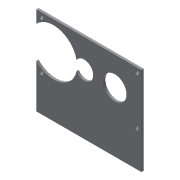
# Autodesk Inventor part: attatching plate for toughbox
Saved by Autodesk Inventor 2015 (Build 190159000, 159)
## iProperties
Created: 2015-02-15
Part Number: attatching plate for toughbox
Material: Generic
Document SubType Name: Sheet Metal
Designer: Noah
Density: 1 g/cm^3
Sheet Metal Rule: Default
Appearance: Default
Author: Noah
Autodesk Inventor part; units mm, degrees
ref_plane "YZ Plane" through (0, 0, 0) normal (1, 0, 0) x (0, 1, 0)
ref_plane "XZ Plane" through (0, 0, 0) normal (0, 1, 0) x (-1, 0, 0)
ref_plane "XY Plane" through (0, 0, 0) normal (0, 0, 1) x (1, 0, 0)
sketch "Sketch1" plane through (0, 0, 0) normal (0, 0, 1) x (1, 0, 0)
  line L0 (0, 0) -> (139.7, 0)
  line L1 (139.7, 0) -> (139.7, 117.475)
  line L2 (139.7, 117.475) -> (0, 117.475)
  line L3 (0, 117.475) -> (0, 0)
  dimension "d0" = 139.7
  dimension "d1" = 117.475
  measures "d0" distance of L2.end L1.end
  measures "d1" distance of L0.end L1.end
extrude "Plate3" add sketch "Sketch1" along normal blind 3.048
sketch "Sketch4" plane through (0, 0, 0) normal (0, 0, -1) x (-1, 0, 0)
  circle A0 centre (-22.86, 79.375) radius 31.242
  circle A1 centre (-6.35, 111.125) radius 2.5527
  circle A2 centre (-6.35, 47.625) radius 2.5527
  circle A3 centre (-133.35, 111.125) radius 2.5527
  circle A4 centre (-133.35, 47.625) radius 2.5527
  arc A5 (-136.4869, 13.4874) -> (-136.4869, 27.7876) centre (-136.4869, 20.6375) ccw
  line L0 (-150.7617, 27.7876) -> (-136.4869, 27.7876)
  line L1 (-136.4869, 13.4874) -> (-150.7617, 13.4874)
  arc A6 (-99.9617, 27.7876) -> (-99.9617, 13.4874) centre (-99.9617, 20.6375) ccw
  line L2 (-99.9617, 27.7876) -> (-85.6869, 27.7876)
  line L3 (-85.6869, 13.4874) -> (-99.9617, 13.4874)
  arc A7 (-85.6869, 13.4874) -> (-85.6869, 27.7876) centre (-85.6869, 20.6375) ccw
  arc A8 (-49.1617, 27.7876) -> (-49.1617, 13.4874) centre (-49.1617, 20.6375) ccw
  line L4 (-49.1617, 27.7876) -> (-34.8869, 27.7876)
  arc A9 (-34.8869, 13.4874) -> (-34.8869, 27.7876) centre (-34.8869, 20.6375) ccw
  line L5 (-34.8869, 13.4874) -> (-49.1617, 13.4874)
  arc A10 (1.6383, 27.7876) -> (1.6383, 13.4874) centre (1.6383, 20.6375) ccw
  line L6 (1.6383, 27.7876) -> (15.9131, 27.7876)
  line L7 (15.9131, 13.4874) -> (1.6383, 13.4874)
  arc A11 (15.9131, 13.4874) -> (15.9131, 27.7876) centre (15.9131, 20.6375) ccw
  circle A12 centre (-104.2924, 79.375) radius 15.5575
  circle A13 centre (-63.5762, 79.375) radius 12.095
  circle A14 centre (-22.86, 79.375) radius 31.242
  circle A15 centre (-6.35, 47.625) radius 2.5527
  circle A16 centre (-63.5762, 79.375) radius 12.095
  circle A17 centre (-104.2924, 79.375) radius 15.5575
  circle A18 centre (-133.35, 111.125) radius 2.5527
  circle A19 centre (-133.35, 47.625) radius 2.5527
  circle A20 centre (-6.35, 111.125) radius 2.5527
  point P0 (0, 0)
  constraints: 21 centre point, 16 end point, 14 point on circle, 8 horizontal, 7 coincident, 7 concentric, 44 other
extrude "Cut1" cut sketch "Sketch4" against normal blind 3.048 contours A0 A13 | A13 A0 | A0 A13 | A1 | A2 | A3 | A4 | A12
equation "\"d12\" = Thickness"
equation "\"BendRadius\" = Thickness"
equation "\"BendReliefWidth\" = Thickness"
equation "\"BendReliefDepth\" = 0.5 * Thickness"
equation "\"CornerReliefSize\" = 4 * Thickness"
equation "\"MinimumRemnant\" = 2 * Thickness"
equation "\"TransitionRadius\" = BendRadius"
equation "\"JacobiRadiusSize\" = BendRadius"
equation "\"GapSize\" = Thickness"
equation "\"d2\" = BendRadius"
equation "\"d3\" = BendRadius"
equation "\"d4\" = BendRadius"
equation "\"Thickness\" = 3.048"
body "Solid3"
